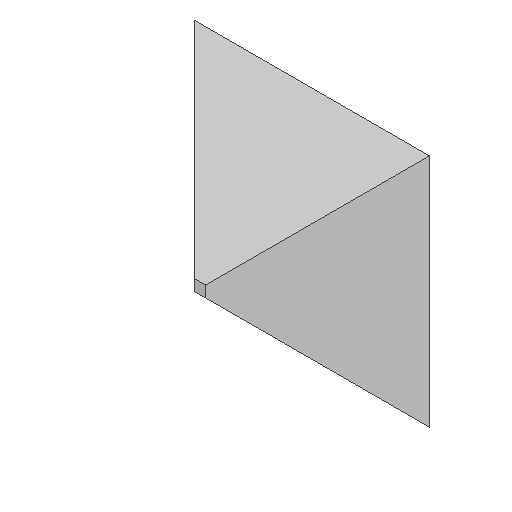
# Autodesk Inventor part: runway
Saved by Autodesk Inventor 2025.2 (Build 292293000, 293)
## iProperties
Created: 2025-08-20
Part Number: runway
Material: Generic
Document SubType Name: Modeling
Designer: user
Density: 1 g/cm^3
Appearance: Default
Author: user
Autodesk Inventor part; units mm, degrees
ref_plane "YZ Plane" through (0, 0, 0) normal (1, 0, 0) x (0, 1, 0)
ref_plane "XZ Plane" through (0, 0, 0) normal (0, 1, 0) x (-1, 0, 0)
ref_plane "XY Plane" through (0, 0, 0) normal (0, 0, 1) x (1, 0, 0)
sketch "Sketch1" plane through (0, 0, 0) normal (0, 1, 0) x (-1, 0, 0)
  line L0 (0.5, 0.5) -> (-0.5, 0.5)
  line L1 (-0.5, 0.5) -> (-0.5, -0.5)
  line L2 (-0.5, -0.5) -> (0.5, -0.5)
  line L3 (0.5, -0.5) -> (0.5, 0.5)
  point P0 (0, 0)
  point P1 (0.5, 0)
  point P2 (0, 0.5)
  dimension "d0" = 1
  dimension "d1" = 1
  constraints: 8 end point, 2 midpoint, 2 parallel, 1 horizontal, 1 horizontal alignment, 1 perpendicular, 1 vertical alignment
  measures "d0" distance of L2.end L1.end
  measures "d1" distance of L1.end L0.end
extrude "Extrusion1" add sketch "Sketch1" against normal blind 10 draft 45
move or copy body "Move Body1" bodies to move or copy 1 copy no rotation origin (0, 0, 0) rotation axis (1, 0, 0) rotation angle 90
